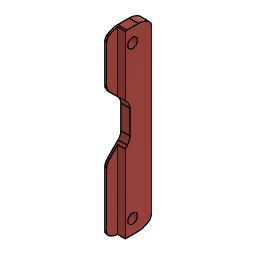
Mobius4_FrameSpacer (Autodesk Fusion 360 design; units mm, degrees)
Autodesk Fusion 360 part; units mm, degrees
sketch "Sketch1" plane through (1.5, 0, 0) normal (1, 0, 0) x (0, 1, 0)
  circle A0 centre (8.8364, -33.427) radius 2.35
  circle A1 centre (-17.5364, -33.427) radius 2.35
  circle A2 centre (4.35, 18.4894) radius 2.35
  circle A3 centre (-11.6364, 31.8073) radius 3.1
  circle A4 centre (0, 0) radius 7.625
  circle A5 centre (-13.65, 11.3596) radius 2.35
  arc A6 (-19.8891, -20.4548) -> (-21.2364, -23.7075) centre (-16.6364, -23.7075) ccw
  line L0 (-21.2364, -23.7075) -> (-21.2364, -53.2005)
  arc A7 (-21.2364, -53.2005) -> (-20.2104, -55.2699) centre (-18.6364, -53.2005) ccw
  arc A8 (-20.2104, -55.2699) -> (-14.7014, -57.127) centre (-14.7014, -48.027) ccw
  line L1 (-14.7014, -57.127) -> (-8.5715, -57.127)
  arc A9 (-8.5715, -57.127) -> (-3.0624, -55.2699) centre (-8.5715, -48.027) ccw
  arc A10 (-3.0624, -55.2699) -> (-2.0364, -53.2005) centre (-4.6364, -53.2005) ccw
  line L2 (-2.0364, -53.2005) -> (-2.0364, -47.4819)
  arc A11 (2.9307, -42.0993) -> (-2.0364, -47.4819) centre (3.3636, -47.4819) ccw
  arc A12 (2.9307, -42.0993) -> (8.2731, -39.657) centre (2.2413, -33.527) ccw
  arc A13 (8.2731, -39.657) -> (15.0041, -30.6101) centre (-17.5364, -13.427) ccw
  arc A14 (15.0041, -30.6101) -> (15.5364, -28.4621) centre (10.9364, -28.4621) ccw
  line L3 (15.5364, -28.4621) -> (15.5364, 15.405)
  arc A15 (15.5364, 15.405) -> (13.7181, 18.5908) centre (11.8364, 15.405) ccw
  arc A16 (13.7181, 18.5908) -> (1.812, 23.8006) centre (-13.65, -27.7449) ccw
  arc A17 (-2.0364, 28.9729) -> (1.812, 23.8006) centre (3.3636, 28.9729) ccw
  line L4 (-2.0364, 28.9729) -> (-2.0364, 34.9809)
  arc A18 (-2.0364, 34.9809) -> (-3.0624, 37.0503) centre (-4.6364, 34.9809) ccw
  arc A19 (-3.0624, 37.0503) -> (-8.5715, 38.9073) centre (-8.5715, 29.8073) ccw
  line L5 (-8.5715, 38.9073) -> (-14.7014, 38.9073)
  arc A20 (-14.7014, 38.9073) -> (-20.2104, 37.0503) centre (-14.7014, 29.8073) ccw
  arc A21 (-20.2104, 37.0503) -> (-21.2364, 34.9809) centre (-18.6364, 34.9809) ccw
  line L6 (-21.2364, 34.9809) -> (-21.2364, 14.7703)
  arc A22 (-21.2364, 14.7703) -> (-19.8891, 11.5176) centre (-16.6364, 14.7703) ccw
  line L7 (-19.8891, 11.5176) -> (-14.1816, 5.8101)
  arc A23 (-12.6, 1.9917) -> (-14.1816, 5.8101) centre (-18, 1.9917) ccw
  line L8 (-12.6, 1.9917) -> (-12.6, -10.9289)
  arc A24 (-14.1816, -14.7473) -> (-12.6, -10.9289) centre (-18, -10.9289) ccw
  line L9 (-14.1816, -14.7473) -> (-19.8891, -20.4548)
  circle A25 centre (-11.6364, -50.027) radius 3.1
  circle A26 centre (-11.6364, 31.8073) radius 2.6
  circle A27 centre (-11.6364, -50.027) radius 2.6
  line L10 (-1.6364, 34.9809) -> (-1.6364, -53.2005)
  line L11 (-8.5715, -57.527) -> (-14.7014, -57.527)
  line L12 (-14.7014, 39.3073) -> (-8.5715, 39.3073)
  line L13 (-8.5715, 39.3073) -> (-14.7014, 39.3073)
  line L14 (-21.6364, 14.7703) -> (-21.6364, 34.9809)
  line L15 (-21.6364, 34.9809) -> (-21.6364, 14.7703)
  line L16 (-13, -10.9289) -> (-13, 1.9917)
  line L17 (-13, 1.9917) -> (-13, -10.9289)
  line L18 (-8.5715, -57.527) -> (-14.7014, -57.527)
  line L19 (-14.7014, -57.527) -> (-8.5715, -57.527)
  line L20 (-1.6364, 34.9809) -> (-1.6364, 28.9729)
  line L21 (-1.6364, 28.9729) -> (-1.6364, 34.9809)
  line L22 (-21.6364, -53.2005) -> (-21.6364, -23.7075)
  line L23 (-21.6364, -23.7075) -> (-21.6364, -53.2005)
  line L24 (-14.4645, 5.5273) -> (-20.172, 11.2347)
  line L25 (-20.172, 11.2347) -> (-14.4645, 5.5273)
  line L26 (-20.172, -20.172) -> (-14.4645, -14.4645)
  line L27 (-14.4645, -14.4645) -> (-20.172, -20.172)
  arc A28 (-21.6364, 14.7703) -> (-20.172, 11.2347) centre (-16.6364, 14.7703) ccw
  arc A29 (-13, 1.9917) -> (-14.4645, 5.5273) centre (-18, 1.9917) ccw
  arc A30 (-14.4645, -14.4645) -> (-13, -10.9289) centre (-18, -10.9289) ccw
  arc A31 (-20.172, -20.172) -> (-21.6364, -23.7075) centre (-16.6364, -23.7075) ccw
  arc A32 (-20.4526, 37.3687) -> (-21.6364, 34.9809) centre (-18.6364, 34.9809) ccw
  arc A33 (-20.4526, 37.3687) -> (-21.6364, 34.9809) centre (-18.6364, 34.9809) ccw
  arc A34 (-14.7014, 39.3073) -> (-20.4526, 37.3687) centre (-14.7014, 29.8073) ccw
  arc A35 (-14.7014, 39.3073) -> (-20.4526, 37.3687) centre (-14.7014, 29.8073) ccw
  arc A36 (-2.8203, 37.3687) -> (-8.5715, 39.3073) centre (-8.5715, 29.8073) ccw
  arc A37 (-2.8203, 37.3687) -> (-8.5715, 39.3073) centre (-8.5715, 29.8073) ccw
  arc A38 (-1.6364, 34.9809) -> (-2.8203, 37.3687) centre (-4.6364, 34.9809) ccw
  arc A39 (-1.6364, 34.9809) -> (-2.8203, 37.3687) centre (-4.6364, 34.9809) ccw
  arc A40 (-2.8203, -55.5883) -> (-1.6364, -53.2005) centre (-4.6364, -53.2005) ccw
  arc A41 (-2.8203, -55.5883) -> (-1.6364, -53.2005) centre (-4.6364, -53.2005) ccw
  arc A42 (-8.5715, -57.527) -> (-2.8203, -55.5883) centre (-8.5715, -48.027) ccw
  arc A43 (-20.4526, -55.5883) -> (-14.7014, -57.527) centre (-14.7014, -48.027) ccw
  arc A44 (-20.4526, -55.5883) -> (-14.7014, -57.527) centre (-14.7014, -48.027) ccw
  arc A45 (-21.6364, -53.2005) -> (-20.4526, -55.5883) centre (-18.6364, -53.2005) ccw
  arc A46 (-21.6364, -53.2005) -> (-20.4526, -55.5883) centre (-18.6364, -53.2005) ccw
  line L28 (-15.6364, 39.2612) -> (-15.6364, -57.4808)
  dimension "d1" = 5.2
  dimension "d2" = 5.2
  dimension "d11" = 4
  constraint concentric A3 A26
  constraint concentric A25 A27
  constraint vertical L10
  constraint horizontal L11
  constraint collinear L11 L18
  constraint collinear L10 L21
  constraint coincident L24.end L25.start
  constraint coincident L14.start L15.end
  constraint coincident L16.end L17.start
  constraint coincident L24.start L25.end
  constraint tangent L24 A29
  constraint coincident L26.end L27.start
  constraint coincident L16.start L17.end
  constraint tangent L16 A30
  constraint coincident L22.end L23.start
  constraint coincident L26.start L27.end
  constraint tangent L26 A31
  constraint tangent L24 A28
  constraint parallel L10 L28
  constraint coincident A34 L28.start
  constraint coincident A43 L28.end
  measures "d1" diameter of A26
  measures "d2" diameter of A27
  measures "d11" distance of A3.centre L28
extrude "Extrude1" add sketch "Sketch1" along normal blind 5 contours A1 L28 | A1 A4 A5 A8 L1 A9 A10 L2 A11 A17 L4 A18 A19 L5 A20 L7 A23 L8 A24 L9 L10 L28 | L7 A23 L8 A24 L9 L16 L17 L24 L25 L26 L27 A29 A30 L28 | A8 L1 A9 A10 L2 A11 L10 L11 L18 L19 A40 A41 A42 A43 A44 L28 | A5 L28 | A17 L4 A18 A19 L5 A20 L10 L12 L13 L20 L21 A34 A35 A36 A37 A38 A39 L28 | A4 L10 | A3 | A25 picked at (-15.5836, -33.8048) picked at (-14.306, 10.6703) picked at (-3.8201, 0.9896)
extrude "Extrude2" add sketch "Sketch1" along normal blind 1 contours A1 L28 | A1 A6 L0 A7 A8 L9 L28 | A6 L0 A7 A8 L9 L22 L23 L26 L27 A31 A43 A44 A45 A46 L28 | A20 A21 L6 A22 L7 L14 L15 L24 L25 A28 A32 A33 A34 A35 L28 | A5 A20 A21 L6 A22 L7 L28 | A5 L28 picked at (-17.0446, -33.3116) picked at (-15.6886, 11.681)
chamfer "Chamfer1" distance 0.4 angle 45 2 edges at (1.5, -14.0605, -49.0868) (1.5, -14.0605, 32.7475)
equation "d2 = d1"
named bodies: "FrameSpacer"
